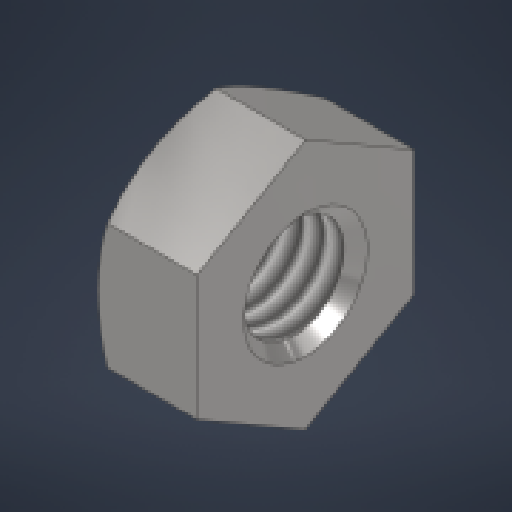
# Autodesk Inventor part: SLBNR4
Saved by Autodesk Inventor 2024 (Build 280153000, 153)
## iProperties
Category: PARTsolutions
Company: MISUMI
Created: 2024-01-28
Part Number: SLBNR4
Material: 스테인리스스틸
Catalog Web Link: www.cadenas.de
Description: LBNR, LBNL, SLBNR, SLBNL, KNTR, KNTL, SKNTR-Nuts
Vendor: MISUMI
Document SubType Name: Modeling
Designer: psAdmin
Manufacturer: MISUMI
Mass: 0.85942 g
Surface Area: 1.72411 cm^2
Volume: 0.107428 cm^3
Density: 8 g/cm^3
Appearance: 반연마
PSOL_IDENT_0: {$CADENAS_DATA/23d-libs/misumi/metric/27_screws_nuts/slbnl.prj},199 {VTYP=3D},{NB=SLBNR4},{LINA=SLBN
PSOL_IDENT_1: R4},{NN=LBNR, LBNL, SLBNR, SLBNL, KNTR, KNTL, SKNTR},{DATE=03.06.2021 03:35:45},{GEOMDATE=05.11.2010
PSOL_IDENT_2: 00:00:00},{VERSION=},{LINEID=30},{WBVAR=TRS,MAT,CS},{WBNUMERIC=}  {NB=SLBNR4},{LINA=SLBNR4},{KT=DUM
PSOL_IDENT_3: MY},{PN=SLBNR4},{TS=LBN},{TRS=R},{MAT=S},{ST=-},{CS=1},{M1=4},{M=4.0},{P=0.70},{B=7.0},{EE=8.1},{T=3
PSOL_IDENT_4: .2},{T1=0.0},{TFX=3.2},{T1FX=2.4},{CALG='1','JIS Class 1','2','JIS Class 3'},{TRSALG= 'R', 'Right-Ha
PSOL_IDENT_5: nd Thread', 'L', 'Left-Hand Thread' },{MATALG= '', 'SWCH Carbon Steel', 'S', '304 Stainless Steel' }
NB: SLBNR4
NN: LBNR, LBNL, SLBNR, SLBNL, KNTR, KNTL, SKNTR
NT: Nuts
NBSYN: $PN.
LINA: SLBNR4
CATALOG: Misumi
PN: SLBNR4
TRS: Right-Hand Thread
MAT: 304 Stainless Steel Equivalent
ST: -
CS: JIS Class 1
M1: 4
P: 0.7
B: 7
EE: 8.1
T: 3.2
T1: 0
SUPPLIER: MISUMI
ARTICLENO: SLBNR4
BOMINFO: SLBNR4
CREATOR: CADENAS GmbH
Title: SLBNR4
Author: Cadenas PARTsolutions
Comments: Nuts
Autodesk Inventor part; units mm, degrees
sketch "Sketch_1" plane through (0, 0, 0) normal (0, 0, 1) x (1, 0, 0)
  line L0 (1.6, 0) -> (-1.6, 0)
  line L1 (-1.6, 0) -> (-1.6, 3.5)
  line L2 (-1.6, 3.5) -> (-1.2825, 4.05)
  line L3 (-1.2825, 4.05) -> (1.6, 4.05)
  line L4 (1.6, 4.05) -> (1.6, 0)
  line L5 (1.6, 0) -> (-1.6, 0)
  constraints: 12 end point
revolve "Revolution1" add sketch "Sketch_1" angle 360 about axis through (1.6, 0, 0) along (1, 0, 0)
sketch "Sketch_2" plane through (0, 0, 0) normal (0, 0, 1) x (1, 0, 0)
  line L0 (1.6, 0) -> (-1.6, 0)
  line L1 (-1.6, 0) -> (-1.6, 2)
  line L2 (-1.6, 2) -> (-1.221, 1.621)
  line L3 (-1.221, 1.621) -> (1.221, 1.621)
  line L4 (1.221, 1.621) -> (1.6, 2)
  line L5 (1.6, 2) -> (1.6, 0)
  line L6 (1.6, 0) -> (-1.6, 0)
  constraints: 14 end point
revolve "Revolution2" cut sketch "Sketch_2" angle 360 about axis through (1.6, 0, 0) along (1, 0, 0)
thread "Thread1" size "M4x0.7" class "6H" standard "ISO Metric profile" full length
sketch "Sketch_3" plane through (0, 0, 0) normal (1, 0, 0) x (0, 1, 0)
  line L0 (-7, 7) -> (-7, -7)
  line L1 (-7, -7) -> (7, -7)
  line L2 (7, -7) -> (7, 7)
  line L3 (7, 7) -> (-7, 7)
  line L4 (-2.0207, 3.5) -> (-4.0415, 0)
  line L5 (-4.0415, 0) -> (-2.0207, -3.5)
  line L6 (-2.0207, -3.5) -> (2.0207, -3.5)
  line L7 (2.0207, -3.5) -> (4.0415, 0)
  line L8 (4.0415, 0) -> (2.0207, 3.5)
  line L9 (2.0207, 3.5) -> (-2.0207, 3.5)
  constraints: 20 end point
extrude "Extrusion1" cut sketch "Sketch_3" along normal mid plane 3.2
ref_plane "cp_XY" through (1.6, 0, 0) normal (1, 0, 0) x (0, 0, -1)
ref_plane "cp_YZ" through (1.6, 0, 0) normal (0, 0, -1) x (0, 1, 0)
ref_plane "cp_ZX" through (1.6, 0, 0) normal (0, 1, 0) x (1, 0, 0)
ref_plane "nut_to_screw_XY" through (0, 0, 0) normal (1, 0, 0) x (0, 0, -1)
ref_plane "nut_to_screw_YZ" through (0, 0, 0) normal (0, 0, -1) x (0, 1, 0)
ref_plane "nut_to_screw_ZX" through (0, 0, 0) normal (0, 1, 0) x (1, 0, 0)
body "Solid1"
